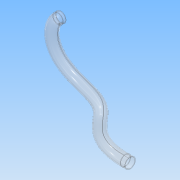
# Autodesk Inventor part: Top_Front Pipe 12
Saved by Autodesk Inventor 2018.1 (Build 221171000, 171)
## iProperties
Created: 2019-03-21
Part Number: Top_Front Pipe 12
Material: PMMA Plastic
Document SubType Name: Modeling
Designer: James
Density: 1.188 g/cm^3
Appearance: Polycarbonate - Clear
Author: James
Autodesk Inventor part; units mm, degrees
ref_plane "YZ Plane" through (0, 0, 0) normal (1, 0, 0) x (0, 1, 0)
ref_plane "XZ Plane" through (0, 0, 0) normal (0, 1, 0) x (-1, 0, 0)
ref_plane "XY Plane" through (0, 0, 0) normal (0, 0, 1) x (1, 0, 0)
sketch "Sketch1" plane through (0, 0, 0) normal (0, 1, 0) x (-1, 0, 0)
  circle A0 centre (0, 0) radius 23
  circle A1 centre (0, 0) radius 20
  dimension "d0" = 3
  dimension "d1" = 40
  constraints: 2 centre point, 2 coincident
  measures "d0" radial gap between concentric circles of A0 A1
  measures "d1" diameter of A1
extrude "Extrusion1" add sketch "Sketch1" along normal blind 12
sketch "Sketch2" plane through (0, 0, 0) normal (0, 0, 1) x (1, 0, 0)
  line L0 (23, 12) -> (-23, 12) projected
  point P0 (0, 0)
  point P1 (0, 5)
  point P2 (0, 12)
  dimension "d4" = 7
  constraints: 1 midpoint, 1 vertical alignment
  measures "d4" distance from line of L0 point (0, 5)
hole "Hole1" at (0, 5, 0) direction (0, 0, -1) diameter 4.5 end through all
sketch "Sketch3" plane through (0, 0, 0) normal (0, -1, 0) x (1, 0, 0)
  circle A0 centre (0, 0) radius 20 projected
  circle A1 centre (0, 0) radius 23 projected
sketch3d "3D Sketch1"
  spline S0 degree 4 poles (0, 0, 0) (0, -40, 0) (0, -40, -150) (292.5, -40, -150) (292.5, -124, -150) (292.5, -124, -256) (412.5, -124, -256) knots 1 1 1 1 1 2 3 4 4 4 4 4
  dimension "d26" = 40
  dimension "d27" = 150
  dimension "d28" = 292.5
  dimension "d29" = 84
  dimension "d30" = 106
  dimension "d31" = 120
sweep "Sweep1" add profiles "Sketch3" path "3D Sketch1"
sketch "Sketch4" plane through (412.5, -124, -256) normal (1, 0, 0) x (0, 0, -1)
  spline S0 degree 6 poles (-19.6738, -3.5977) (-25.6514, 29.0911) (13.911, 41.1763) (54.0855, 9.8904) (27.5829, -33.5884) (-13.6961, -36.2865) (-19.6738, -3.5977) knots 0 0 0 0 0 0 0 1 1 1 1 1 1 1 weights 1.669078 1.03673 1.038347 0.853534 1.038347 1.03673 1.669078 projected
  circle A0 centre (0, 0) radius 23 projected
  point P0 (-256, 124)
  point P1 (-22.3526, -5.4186)
  constraints: 2 other
extrude "Extrusion2" add sketch "Sketch4" along normal blind 20 contours S0 picked at (-0.7641, 21.8443)
body "Solid1"
